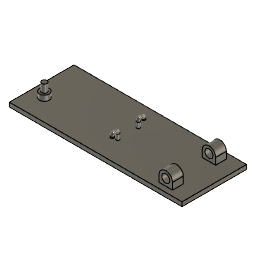
Baza_collective (Autodesk Fusion 360 design; units mm, degrees)
part number: 2026-02-12-14-45-39-089
Autodesk Fusion 360 part; units mm, degrees
note: some values were not read from the file. Set by a fixed rule: which sketch regions a step uses.
sketch "Szkic1" plane through (0, 0, 0) normal (0, 0, 1) x (1, 0, 0)
  line L0 (160, 60) -> (-160, 60)
  line L1 (-160, 60) -> (-160, -60)
  line L2 (-160, -60) -> (160, -60)
  line L3 (160, -60) -> (160, 60)
  line L4 (160, 60) -> (-160, -60) construction
  line L5 (-160, 60) -> (160, -60) construction
  dimension "d1" = 120
  dimension "d2" = 320
  constraint horizontal L0
  constraint perpendicular L0 L1
  constraint parallel L0 L2
  constraint parallel L1 L3
  constraint coincident L4 origin
  constraint coincident L5 origin
  measures "d1" distance of L0.start L2.end
  measures "d2" distance of L0.start L0.end
extrude "Wyciągnięcie proste1" add sketch "Szkic1" along normal blind 8
sketch "Szkic2" plane through (0, 0, 0) normal (0, 1, 0) x (1, 0, 0)
  line L0 (107.5, -8) -> (107.5, -20.5)
  line L1 (107.5, -20.5) -> (132.5, -20.5)
  line L2 (132.5, -20.5) -> (132.5, -8)
  circle A0 centre (120, -20.5) radius 12.5
  line L3 (107.5, -8) -> (132.5, -8)
  line L4 (-160, -8) -> (160, -8)
  circle A1 centre (120, -20.5) radius 7.5
  dimension "d5" = 15
  dimension "d6" = 25
  dimension "d7" = 40
  constraint vertical L0
  constraint perpendicular L0 L1
  constraint perpendicular L1 L2
  constraint midpoint L1 A0.centre
  constraint coincident L1.end A0
  constraint perpendicular L0 L3
  constraint collinear L3 L4
  constraint concentric A0 A1
  constraint tangent A0 L3
  measures "d5" diameter of A1
  measures "d6" diameter of A0
  measures "d7" horizontal distance of L4.end A0.centre
extrude "Wyciągnięcie proste2" add sketch "Szkic2" against normal blind 20 from surface at 50 contours L0 A0 L3 L4 | L1 A0 A1 | L1 A0 A1 | L2 A0 L3 L4
sketch "Szkic4" plane through (0, 0, 0) normal (1, 0, 0) x (0, 1, 0)
  line L0 (19, 8) -> (19, 18)
  arc A0 (24, 23) -> (19, 18) centre (24, 18) ccw
  line L1 (29, 18) -> (29, 16)
  arc A1 (29, 18) -> (24, 23) centre (24, 18) ccw
  point P0 (19, 23)
  point P1 (29, 23)
  dimension "d11" = 15
  dimension "d12" = 10
  dimension "d13" = 5
  dimension "d23" = 7
  dimension "d24" = 5
  constraint vertical L0
  constraint coincident P0 L0
  constraint tangent L0 A0
  constraint coincident P1 L1
  constraint tangent L1 A1
  constraint coincident A0.start A1.end
  measures "d11" distance of L0.start P0
  measures "d12" distance of P0 P1
  measures "d13" radius of A0
  measures "d23" distance of P1 L1.end
  measures "d24" radius of A1
ref_plane "Płaszczyzna konstrukcyjna1" through (0, 29, 0) normal (0, 1, 0) x (0, 0, 1)
sketch "Szkic6" plane through (0, 0, 8) normal (0, 0, 1) x (-1, 0, 0)
  circle A0 centre (0, -19) radius 3
  circle A1 centre (0, -19) radius 5
  line L0 (-132.5, -50) -> (-132.5, -30)
  line L1 (-132.5, -30) -> (-107.5, -30)
  line L2 (-107.5, -30) -> (-107.5, -50)
  line L3 (-107.5, -50) -> (-132.5, -50)
  line L4 (-160, 60) -> (-160, -60)
  line L5 (-160, -60) -> (160, -60)
  line L6 (160, -60) -> (160, 60)
  line L7 (160, 60) -> (-160, 60)
  point P0 (0, -19)
  dimension "d14" = 10
  dimension "d15" = 6
  constraint concentric A0 A1
  constraint coincident P0 A0.centre
  measures "d14" diameter of A1
  measures "d15" diameter of A0
sweep "Przeciągnięcie2" add profiles "Szkic6" path "Szkic4" along L1 A1 A0 L0 section 1 contours A0
mirror "Odbij1" about plane through (0, 0, 0) normal (0, 1, 0) of "Wyciągnięcie proste2", "Przeciągnięcie2"
sketch "Szkic7" plane through (0, 0, 8) normal (0, 0, 1) x (-1, 0, 0)
sketch "Szkic8" plane through (0, 0, 8) normal (0, 0, 1) x (-1, 0, 0)
  circle A0 centre (135, 20) radius 5
  line L0 (160, -60) -> (160, 60)
  line L1 (-160, -60) -> (160, -60)
  line L2 (0, 0) -> (60, 0)
  circle A1 centre (135, 20) radius 9
  dimension "d33" = 10
  dimension "d34" = 25
  dimension "d38" = 80
  dimension "d39" = 18
  constraint coincident L2.start origin
  constraint horizontal L2
  constraint concentric A0 A1
  measures "d33" diameter of A0
  measures "d34" distance of A0.centre L0
  measures "d38" distance of A0.centre L1
  measures "d39" diameter of A1
extrude "Wyciągnięcie proste3" add sketch "Szkic8" along normal blind 10 contours A0 | A1
extrude "Wyciągnięcie proste4" add sketch "Szkic8" along normal blind 25 contours A0
